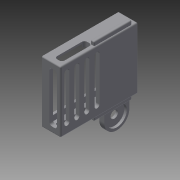
# Autodesk Inventor part: 160729 T_TH_P_Box_R23
Saved by Autodesk Inventor 2015 (Build 190159000, 159)
## iProperties
Created: 2015-12-10
Part Number: 160729 T_TH_P_Box_R23
Material: Generico
Document SubType Name: Modeling
Designer: piscian
Density: 1 g/cm^3
Appearance: Default
Author: piscian
Autodesk Inventor part; units mm, degrees
sketch "Schizzo1" plane through (0, 0, 0) normal (0, 0, 1) x (1, 0, 0)
  line L0 (-10.75, 0) -> (10.25, 0)
  line L1 (-9.2967, 5) -> (-11.45, 5)
  line L2 (-11.45, 5) -> (-11.45, 3)
  line L3 (-11.45, 3) -> (-10.75, 3)
  line L4 (10.25, 5) -> (11.45, 5)
  line L5 (11.45, 5) -> (11.45, 3)
  line L6 (11.45, 3) -> (10.25, 3)
  line L7 (-9.2967, 6) -> (-9.2967, 5)
  line L8 (-10.75, 3) -> (-10.75, 0)
  line L9 (10.25, 0) -> (10.25, 3)
  line L10 (10.25, 5) -> (10.25, 6)
  line L11 (-9.2967, 6) -> (-12.2967, 6)
  line L12 (-12.2967, 6) -> (-12.2967, -1.5)
  line L13 (-12.2967, -1.5) -> (12.25, -1.5)
  line L14 (12.25, -1.5) -> (12.25, 6)
  line L15 (12.25, 6) -> (10.25, 6)
  point P0 (0, 0)
  dimension "d0" = 21
  dimension "d3" = 22.9
  dimension "d4" = 11.45
  dimension "d5" = 3
  dimension "d6" = 0
  dimension "d7" = 3
  dimension "d8" = 2
  dimension "d9" = 2
  dimension "d12" = 1.5
  dimension "d13" = 2
  dimension "d14" = 3
  dimension "d17" = 1
  dimension "d18" = 1
  dimension "d112" = 2
  constraints: 32 end point, 4 parallel, 3 horizontal, 3 perpendicular, 1 collinear
  measures "d0" distance of L0.start L0.end
  measures "d3" distance between parallel lines of L5 L2
  measures "d4" distance from line of point (0, 0) L2
  measures "d5" distance between parallel lines of L3 L0
  measures "d6" distance from line of point (0, 0) L0
  measures "d7" distance between parallel lines of L0 L6
  measures "d8" distance between parallel lines of L6 L4
  measures "d9" distance of L1.end L2.end
  measures "d12" distance between parallel lines of L0 L13
  measures "d13" distance between parallel lines of L14 L9
  measures "d14" distance of L7.start L11.end
  measures "d17" distance between parallel lines of L15 L4
  measures "d18" distance between parallel lines of L11 L1
  measures "d112" distance between parallel lines of L14 L10
extrude "Body" add sketch "Schizzo1" along normal blind 26.9
sketch "Schizzo2" plane through (0, 0, 26.9) normal (0, 0, 1) x (1, 0, 0)
  line L0 (-12.2967, 6) -> (12.25, 6)
  line L1 (12.25, 6) -> (12.25, -1.5)
  line L2 (12.25, -1.5) -> (-12.2967, -1.5)
  line L3 (-12.2967, -1.5) -> (-12.2967, 6)
  point P0 (0, 0)
  constraints: 8 end point, 2 parallel, 1 horizontal, 1 perpendicular
extrude "Closure" add sketch "Schizzo2" along normal blind 1.5
sketch "Schizzo4" plane through (0, 0, 0) normal (0, 0, -1) x (-1, 0, 0)
  line L0 (10.75, 0) -> (-10.25, 0) projected
  line L1 (-10.25, 0) -> (-10.25, 3) projected
  line L2 (-10.25, 3) -> (-11.45, 3) projected
  line L3 (-11.45, 3) -> (-11.45, 5) projected
  line L4 (-11.45, 5) -> (-10.25, 5) projected
  line L5 (-10.25, 5) -> (-10.25, 6) projected
  line L6 (-10.25, 6) -> (-12.25, 6) projected
  line L7 (-12.25, 6) -> (-12.25, -1.5) projected
  line L8 (-12.25, -1.5) -> (12.2967, -1.5) projected
  line L9 (12.2967, -1.5) -> (12.2967, 6) projected
  line L10 (12.2967, 6) -> (9.2967, 6) projected
  line L11 (9.2967, 6) -> (9.2967, 5) projected
  line L12 (9.2967, 5) -> (11.45, 5) projected
  line L13 (11.45, 5) -> (11.45, 3) projected
  line L14 (11.45, 3) -> (10.75, 3) projected
  line L15 (10.75, 3) -> (10.75, 0) projected
  point P0 (0, 0)
extrude "Estrusione3" add sketch "Schizzo4" along normal blind 2.5
ref_plane "Piano di lavoro1" through (0, 0, -1.5) normal (0, 0, -1) x (-1, 0, 0)
sketch "Schizzo5" plane through (0, 0, -1.5) normal (0, 0, -1) x (-1, 0, 0)
  line L0 (-11.45, 6.5) -> (11.45, 6.5)
  line L1 (11.45, 6.5) -> (11.45, -1)
  line L2 (11.45, -1) -> (-11.45, -1)
  line L3 (-11.45, -1) -> (-11.45, 6.5)
  line L4 (12.2967, -1.5) -> (-12.25, -1.5) projected
  point P0 (0, 0)
  dimension "d25" = 22.9
  dimension "d27" = 11.45
  dimension "d28" = 0.5
  dimension "d31" = 8
  constraints: 8 end point, 2 parallel, 1 horizontal, 1 perpendicular
  measures "d25" distance of L1.end L2.end
  measures "d27" distance from line of point (0, 0) L3
  measures "d28" distance between parallel lines of L2 L4
  measures "d31" distance between parallel lines of L0 L4
extrude "Fente de passage fermeture" cut sketch "Schizzo5" against normal blind 1.5
sketch "Schizzo6" plane through (12.25, -1.5, 28.4) normal (1, 0, 0) x (0, 0, -1)
  line L0 (0, 0) -> (0, 7.5) projected
  line L1 (0, 0) -> (30.9, 0) projected
  line L2 (3, 4.5) -> (13, 4.5)
  line L3 (14, 3.5) -> (14, 2.5)
  line L4 (13, 1.5) -> (3, 1.5)
  line L5 (2, 2.5) -> (2, 3.5)
  arc A0 (14, 3.5) -> (13, 4.5) centre (13, 3.5) ccw
  arc A1 (13, 1.5) -> (14, 2.5) centre (13, 2.5) ccw
  arc A2 (2, 2.5) -> (3, 1.5) centre (3, 2.5) ccw
  arc A3 (3, 4.5) -> (2, 3.5) centre (3, 3.5) ccw
  point P0 (28.4, 1.5)
  point P1 (2, 4.5)
  point P2 (14, 1.5)
  point P3 (14, 4.5)
  point P4 (2, 1.5)
  dimension "d36" = 12
  dimension "d37" = 1.5
  dimension "d48" = 2
  dimension "d58" = 3
  dimension "d157" = 1
  constraints: 8 end point, 8 point on circle, 8 point on line, 8 tangent, 4 centre point, 3 equal radius, 2 parallel, 1 horizontal, 1 perpendicular
  measures "d36" distance between parallel lines of L3 L5
  measures "d37" distance between parallel lines of L4 L1
  measures "d48" distance between parallel lines of L5 L0
  measures "d58" distance of point (2, 1.5) point (2, 4.5)
  measures "d157" radius of A0
extrude "Short Air sampling" cut sketch "Schizzo6" against normal blind 30
fillet "Raccordo1" radius 0.5 5 edges at (-0.0233, -1.5, 28.4) (12.25, -1.5, 12.95) (12.25, 2.25, 28.4) (-12.2967, 2.25, 28.4) (-12.2967, -1.5, 12.95)
fillet "Raccordo2" radius 0.5 5 edges at (-12.1502, -1.3536, -2.5) (-12.2967, 2.5, -2.5) (12.1036, -1.3536, -2.5) (12.25, 2.5, -2.5) (-0.0233, -1.5, -2.5)
sketch "Sketch10" plane through (-12.2967, -1, 27.9) normal (-1, 0, 0) x (0, 0, 1)
  line L0 (-28.4, 1.5) -> (-13.4, 1.5)
  line L1 (-13.4, 1.5) -> (-13.4, 0)
  line L2 (-13.4, 0) -> (-28.4, 0)
  line L3 (-28.4, 0) -> (-28.4, 1.5)
  line L4 (-29.9, -0.5) -> (0, -0.5) projected
  line L5 (-30.4, 7) -> (-30.4, 0) projected
  line L6 (0.5, 0) -> (0.5, 7) projected
  point P0 (-27.9, 1)
  dimension "d82" = 15
  dimension "d83" = 1.5
  dimension "d84" = 0.5
  dimension "d113" = 13.9
  constraints: 8 end point, 2 parallel, 1 horizontal, 1 perpendicular
  measures "d82" distance of L1.end L2.end
  measures "d83" distance of L2.end L0.start
  measures "d84" distance between parallel lines of L4 L2
  measures "d113" distance between parallel lines of L1 L6
sketch "Sketch11" plane through (0, 0, 28.4) normal (0, 0, 1) x (1, 0, 0)
  line L0 (8.977, 0) -> (-9.023, 0)
  line L1 (-10.023, 1) -> (-10.023, 2)
  line L2 (-9.023, 3) -> (8.977, 3)
  line L3 (9.977, 2) -> (9.977, 1)
  line L4 (12.25, -1) -> (12.25, 6) projected
  line L5 (-11.7967, -1.5) -> (11.75, -1.5) projected
  line L6 (-12.2967, 6) -> (-12.2967, -1) projected
  arc A0 (-10.023, 1) -> (-9.023, 0) centre (-9.023, 1) ccw
  arc A1 (-9.023, 3) -> (-10.023, 2) centre (-9.023, 2) ccw
  arc A2 (9.977, 2) -> (8.977, 3) centre (8.977, 2) ccw
  arc A3 (8.977, 0) -> (9.977, 1) centre (8.977, 1) ccw
  point P0 (0, 0)
  point P1 (9.977, 0)
  point P2 (-10.023, 3)
  point P3 (-10.023, 0)
  point P4 (9.977, 3)
  dimension "d85" = 20
  dimension "d86" = 3
  dimension "d87" = 2.273
  dimension "d88" = 1.5
  dimension "d156" = 1
  constraints: 8 end point, 8 point on circle, 8 point on line, 8 tangent, 4 centre point, 3 equal radius, 2 parallel, 1 horizontal, 1 perpendicular
  measures "d85" distance of point (9.977, 0) point (-10.023, 0)
  measures "d86" distance of point (9.977, 3) point (9.977, 0)
  measures "d87" distance between parallel lines of L3 L4
  measures "d88" distance between parallel lines of L0 L5
  measures "d156" radius of A0
extrude "Long Air Sampling" cut sketch "Sketch11" against normal blind 3
extrude "Handle 1" add sketch "Sketch10" along normal blind 1.5
sketch "Sketch12" plane through (12.25, -1, 27.9) normal (1, 0, 0) x (0, 0, -1)
  line L0 (28.4, 0) -> (13.4, 0)
  line L1 (13.4, 0) -> (13.4, 1.5)
  line L2 (13.4, 1.5) -> (28.4, 1.5)
  line L3 (28.4, 1.5) -> (28.4, 0)
  line L4 (0, -0.5) -> (29.9, -0.5) projected
  line L5 (30.4, 0) -> (30.4, 7) projected
  line L6 (-0.5, 7) -> (-0.5, 0) projected
  point P0 (27.9, 1)
  dimension "d102" = 15
  dimension "d103" = 1.5
  dimension "d104" = 0.5
  dimension "d114" = 13.9
  constraints: 8 end point, 2 parallel, 1 horizontal, 1 perpendicular
  measures "d102" distance of L0.start L0.end
  measures "d103" distance of L2.end L0.start
  measures "d104" distance between parallel lines of L0 L4
  measures "d114" distance between parallel lines of L6 L1
extrude "Handle 2" add sketch "Sketch12" along normal blind 1.5
fillet "Fillet Handle 2" radius 0.4 8 edges at (13, 0.5, -0.5) (13, -1, -0.5) (13.75, -0.25, -0.5) (13.75, 0.5, 7) (13.75, -1, 7) (13.75, -0.25, 14.5) (13, 0.5, 14.5) (13, -1, 14.5)
fillet "Fillet Handle 1" radius 0.4 8 edges at (-13.7967, -1, 7) (-13.7967, 0.5, 7) (-13.7967, -0.25, -0.5) (-13.7967, -0.25, 14.5) (-13.0467, -1, 14.5) (-13.0467, 0.5, 14.5) (-13.0467, -1, -0.5) (-13.0467, 0.5, -0.5)
sketch "Sketch13" plane through (-11.7967, -1.5, 27.9) normal (0, -1, 0) x (1, 0, 0)
  line L0 (23.5467, 0) -> (23.5467, -29.9) construction
  line L1 (23.5467, -29.9) -> (0, -29.9) construction
  line L2 (0, -29.9) -> (0, 0) construction
  line L3 (0, 0) -> (23.5467, 0) construction
  line L4 (23.5467, -29.9) -> (0, -29.9) projected
  line L5 (0, 0) -> (0, -29.9) projected
  line L6 (0, 0) -> (23.5467, 0) projected
  line L7 (23.5467, 0) -> (23.5467, -29.9) projected
  point P0 (11.7967, -27.9)
  constraints: 2 coincident, 1 vertical, 2 other
emboss "Emboss1" [suppressed]
sketch "Sketch14" plane through (0, 0, -1.5) normal (0, 0, -1) x (-1, 0, 0)
  line L0 (-10.25, 0) -> (-10.25, 3) projected
  line L1 (-10.25, 1) -> (10.75, 1)
  line L2 (10.75, 1) -> (10.75, 0)
  line L3 (10.75, 0) -> (-10.25, 0)
  line L4 (-10.25, 0) -> (-10.25, 1)
  line L5 (-11.75, -1.5) -> (11.7967, -1.5) projected
  point P0 (0, 0)
  dimension "d115" = 1
  dimension "d124" = 2.5
  constraints: 8 end point, 2 parallel, 1 horizontal, 1 perpendicular, 1 point on line
  measures "d115" distance of L1.end L2.end
  measures "d124" distance between parallel lines of L5 L1
extrude "Guidage fond ext" add sketch "Sketch14" along normal blind 1
ref_plane "Work Plane3" through (-4.6483, 6, 0) normal (0, 0, -1) x (-1, 0, 0)
sketch "Sketch15" plane through (-4.6483, 6, 0) normal (0, 0, -1) x (-1, 0, 0)
  line L0 (6.1017, -6) -> (6.1017, -3) projected
  line L1 (-14.8983, -6.0524) -> (6.1017, -6.0524)
  line L2 (6.1017, -6.0524) -> (6.1017, -5.0524)
  line L3 (6.1017, -5.0524) -> (-14.8983, -5.0524)
  line L4 (-14.8983, -5.0524) -> (-14.8983, -6.0524)
  line L5 (-16.3983, -7.5) -> (7.1483, -7.5) projected
  line L6 (-14.8983, -6) -> (6.1017, -6) projected
  point P0 (-4.6483, -6)
  point P1 (-14.8983, -5)
  dimension "d119" = 1
  dimension "d122" = 2.4476
  dimension "d123" = 0.0524
  constraints: 8 end point, 2 parallel, 1 horizontal, 1 perpendicular
  measures "d119" distance between parallel lines of L3 L1
  measures "d122" distance between parallel lines of L5 L3
  measures "d123" distance between parallel lines of L6 L1
extrude "Guidage fond int." add sketch "Sketch15" against normal blind 1
ref_plane "Work Plane4" through (-12.2967, 3.5157, -2) normal (-1, 0, 0) x (0, -1, 0)
sketch "Sketch16" plane through (-12.2967, 3.5157, -2) normal (-1, 0, 0) x (0, -1, 0)
  line L0 (0.5157, -0.5) -> (-1.4843, -0.5) projected
  line L1 (-0.4843, -0.5) -> (1.5157, -0.5)
  line L2 (1.5157, -0.5) -> (1.5157, 9.5)
  line L3 (1.5157, 9.5) -> (-0.4843, 9.5)
  line L4 (-0.4843, 9.5) -> (-0.4843, -0.5)
  point P0 (3.5157, 2)
  dimension "d125" = 2
  dimension "d126" = 10
  constraints: 8 end point, 2 parallel, 1 horizontal, 1 midpoint, 1 perpendicular
  measures "d125" distance of L3.end L2.end
  measures "d126" distance of L2.end L1.end
extrude "Bride de vissage" add sketch "Sketch16" along normal blind 12
fillet "Fillet6" radius 5 2 edges at (-24.2967, 3, -2.5) (-24.2967, 3, 7.5)
fillet "Fillet7" radius 1.5 1 edges at (-12.2967, 3, 7.5)
ref_plane "Work Plane5" through (-12.2967, 3, -2.5) normal (0, -1, 0) x (1, 0, 0)
sketch "Sketch22" plane through (-12.2967, 3, -2.5) normal (0, -1, 0) x (1, 0, 0)
  circle A0 centre (-7, 5) radius 4
  arc A1 (-7, 10) -> (-7, 0) centre (-7, 5) ccw projected
  point P0 (12.2967, 2.5)
  dimension "d136" = 8
  dimension "d142" = 0
  constraints: 1 centre point
  measures "d136" diameter of A0
  measures "d142" distance of A1.centre A0.centre
extrude "Evasement vis de fixation" cut sketch "Sketch22" along normal blind 1
ref_plane "Work Plane8" through (-11.45, 3, -1.5) normal (0, -1, 0) x (1, 0, 0)
sketch "Sketch23" plane through (-11.45, 3, -1.5) normal (0, -1, 0) x (1, 0, 0)
  arc A0 (-7.8467, 9) -> (-7.8467, -1) centre (-7.8467, 4) ccw projected
  circle A1 centre (-7.8467, 4) radius 1.5
  point P0 (11.45, 1.5)
  dimension "d139" = 3
  constraints: 1 centre point, 1 coincident
  measures "d139" diameter of A1
extrude "Alesage vis de fixation" cut sketch "Sketch23" against normal blind 1
sketch "Sketch24" plane through (-11.7967, -1.5, 27.9) normal (0, -1, 0) x (1, 0, 0)
  line L0 (2.5, -1) -> (2.5, -27.9) projected
  line L1 (21.0467, -1) -> (3.5, -1)
  line L2 (2.5, -2) -> (2.5, -2)
  line L3 (3.5, -3) -> (21.0467, -3)
  line L4 (22.0467, -2) -> (22.0467, -2)
  arc A0 (22.0467, -2) -> (21.0467, -1) centre (21.0467, -2) ccw
  arc A1 (21.0467, -3) -> (22.0467, -2) centre (21.0467, -2) ccw
  arc A2 (2.5, -2) -> (3.5, -3) centre (3.5, -2) ccw
  arc A3 (3.5, -1) -> (2.5, -2) centre (3.5, -2) ccw
  line L5 (21.0467, -5) -> (3.5, -5)
  line L6 (2.5, -6) -> (2.5, -6)
  line L7 (3.5, -7) -> (21.0467, -7)
  line L8 (22.0467, -6) -> (22.0467, -6)
  arc A4 (22.0467, -6) -> (21.0467, -5) centre (21.0467, -6) ccw
  arc A5 (21.0467, -7) -> (22.0467, -6) centre (21.0467, -6) ccw
  arc A6 (2.5, -6) -> (3.5, -7) centre (3.5, -6) ccw
  arc A7 (3.5, -5) -> (2.5, -6) centre (3.5, -6) ccw
  line L9 (21.0467, -9) -> (3.5, -9)
  line L10 (2.5, -10) -> (2.5, -10)
  line L11 (3.5, -11) -> (21.0467, -11)
  line L12 (22.0467, -10) -> (22.0467, -10)
  arc A8 (22.0467, -10) -> (21.0467, -9) centre (21.0467, -10) ccw
  arc A9 (21.0467, -11) -> (22.0467, -10) centre (21.0467, -10) ccw
  arc A10 (2.5, -10) -> (3.5, -11) centre (3.5, -10) ccw
  arc A11 (3.5, -9) -> (2.5, -10) centre (3.5, -10) ccw
  line L13 (21.0467, -13) -> (3.5, -13)
  line L14 (2.5, -14) -> (2.5, -14)
  line L15 (3.5, -15) -> (21.0467, -15)
  line L16 (22.0467, -14) -> (22.0467, -14)
  arc A12 (22.0467, -14) -> (21.0467, -13) centre (21.0467, -14) ccw
  arc A13 (21.0467, -15) -> (22.0467, -14) centre (21.0467, -14) ccw
  arc A14 (2.5, -14) -> (3.5, -15) centre (3.5, -14) ccw
  arc A15 (3.5, -13) -> (2.5, -14) centre (3.5, -14) ccw
  point P0 (11.7967, -27.9)
  point P1 (22.0467, -1)
  point P2 (2.5, -3)
  point P3 (2.5, -1)
  point P4 (22.0467, -5)
  point P5 (2.5, -7)
  point P6 (2.5, -5)
  point P7 (22.0467, -9)
  point P8 (2.5, -11)
  point P9 (2.5, -9)
  point P10 (22.0467, -13)
  point P11 (2.5, -15)
  point P12 (2.5, -13)
  dimension "d144" = 2
  dimension "d145" = 1
  dimension "d146" = 1
  dimension "d151" = 4
  constraints: 32 end point, 32 point on circle, 25 point on line, 16 centre point, 8 tangent, 2 equal radius, 2 parallel, 1 horizontal, 1 perpendicular, 1 vertical, 69 other
  measures "d144" distance of point (2.5, -3) point (2.5, -1)
  measures "d145" radius of A0
  measures "d146" radius of A3
  measures "d151" distance of point (2.5, -3) point (2.5, -7)
extrude "Extrusion16" cut sketch "Sketch24" against normal blind 2
equation "\"d4\" = 0.5 * d3"
equation "\"d5\" = d7"
equation "\"d9\" = d8"
equation "\"d18\" = d17"
equation "\"d27\" = 0.5 * d25"
equation "\"d2\" = 0.5 * d0"
equation "\"d35\" = d32"
equation "\"d32\" = 0.5"
